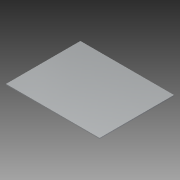
# Autodesk Inventor part: UltibotsGlass230x290
Saved by Autodesk Inventor 2015 SP1 (Build 190203100, 203)
## iProperties
Created: 2014-12-21
Part Number: UltibotsGlass230x290
Material: Glass
Document SubType Name: Modeling
Designer: Jack
Density: 2.18 g/cm^3
Appearance: Clear
Mass: 437.166 g
Surface Area: 1368.13 cm^2
Volume: 200.535 cm^3
Catalog Web Link: http://www.ultibots.com/borosilicate-print-surface-230mm-x-290mm/
Vendor: Ultibots
Author: Jack
Autodesk Inventor part; units mm, degrees
ref_plane "YZ Plane" through (0, 0, 0) normal (1, 0, 0) x (0, 1, 0)
ref_plane "XZ Plane" through (0, 0, 0) normal (0, 1, 0) x (-1, 0, 0)
ref_plane "XY Plane" through (0, 0, 0) normal (0, 0, 1) x (1, 0, 0)
sketch "Sketch1" plane through (0, 0, 0) normal (0, 0, 1) x (1, 0, 0)
  line L0 (0, 0) -> (290, 0)
  line L1 (290, 0) -> (290, 230.5)
  line L2 (290, 230.5) -> (0, 230.5)
  line L3 (0, 230.5) -> (0, 0)
  dimension "d0" = 290
  dimension "d1" = 230.5
  constraints: 8 end point, 2 parallel, 1 horizontal, 1 perpendicular
  measures "d0" distance of L2.end L1.end
  measures "d1" distance of L1.end L0.end
extrude "Extrusion1" add sketch "Sketch1" along normal blind 3
body "Solid1"
